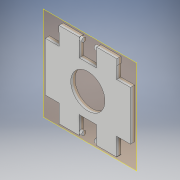
# Autodesk Inventor part: 20_Cube_Insert_focusing_holder_v3
Saved by Autodesk Inventor 2019 (Build 230136000, 136)
## iProperties
Created: 2021-04-22
Part Number: 20_Cube_Insert_focusing_holder_v3
Material: Generic
Document SubType Name: Modeling
Designer: UC2
Density: 1 g/cm^3
Appearance: Default
Author: UC2
Autodesk Inventor part; units mm, degrees
ref_plane "YZ Plane" through (0, 0, 0) normal (1, 0, 0) x (0, 1, 0)
ref_plane "XZ Plane" through (0, 0, 0) normal (0, 1, 0) x (-1, 0, 0)
ref_plane "XY Plane" through (0, 0, 0) normal (0, 0, 1) x (1, 0, 0)
sketch "Skizze1" plane through (0, 0, 0) normal (0, 0, 1) x (1, 0, 0)
  line L0 (0, -42.3366) -> (0, 42.3366) construction
  line L1 (-38.4382, 0) -> (56.3005, 0) construction
  line L2 (0, 0) -> (30.2404, 30.2404) construction
  line L3 (0, 0) -> (42.7664, 0) construction
  line L4 (0, 24.9041) -> (16.9, 24.9041)
  line L5 (16.9, 24.9041) -> (16.9, 21.2841)
  line L6 (16.9, 21.2841) -> (19.092, 19.092)
  line L7 (24.9041, 0) -> (24.9041, 16.9)
  line L8 (24.9041, 16.9) -> (21.2841, 16.9)
  line L9 (21.2841, 16.9) -> (19.092, 19.092)
  line L10 (0, 24.9041) -> (-16.9, 24.9041)
  line L11 (-16.9, 24.9041) -> (-16.9, 21.2841)
  line L12 (-16.9, 21.2841) -> (-19.092, 19.092)
  line L13 (-24.9041, 0) -> (-24.9041, 16.9)
  line L14 (-24.9041, 16.9) -> (-21.2841, 16.9)
  line L15 (-21.2841, 16.9) -> (-19.092, 19.092)
  line L16 (0, 0) -> (30.2404, -30.2404) construction
  line L17 (0, -24.9041) -> (16.9, -24.9041)
  line L18 (16.9, -24.9041) -> (16.9, -21.2841)
  line L19 (16.9, -21.2841) -> (19.092, -19.092)
  line L20 (24.9041, 0) -> (24.9041, -16.9)
  line L21 (24.9041, -16.9) -> (21.2841, -16.9)
  line L22 (21.2841, -16.9) -> (19.092, -19.092)
  line L23 (0, -24.9041) -> (-16.9, -24.9041)
  line L24 (-16.9, -24.9041) -> (-16.9, -21.2841)
  line L25 (-16.9, -21.2841) -> (-19.092, -19.092)
  line L26 (-24.9041, 0) -> (-24.9041, -16.9)
  line L27 (-24.9041, -16.9) -> (-21.2841, -16.9)
  line L28 (-21.2841, -16.9) -> (-19.092, -19.092)
  circle A0 centre (0, 0) radius 10
  dimension "d0" = 45
  dimension "d1" = 16.9
  dimension "d2" = 3.1
  dimension "d3" = 3.62
  dimension "d4" = 20
  constraints: 54 end point, 21 symmetric about line, 3 point on line, 2 horizontal, 2 perpendicular, 1 centre point, 1 coincident, 1 equal length
  measures "d0" angle of L3 L2
  measures "d1" distance of L4.start L4.end
  measures "d2" distance of L5.end L6.end
  measures "d3" distance of L4.end L5.end
  measures "d4" diameter of A0
extrude "Extrusion1" add sketch "Skizze1" along normal blind 2.5
sketch "Skizze2" plane through (0, 0, 2.5) normal (0, 0, 1) x (1, 0, 0)
  line L0 (17.3243, 16.97) -> (5, 16.97) construction
  line L1 (17.3243, 16.97) -> (17.3243, 14.47) construction
  line L2 (5, 14.47) -> (17.3243, 14.47) construction
  line L3 (5, 16.97) -> (5, 14.47) construction
  line L4 (-5, 16.97) -> (-17.3243, 16.97) construction
  line L5 (-5, 16.97) -> (-5, 14.47) construction
  line L6 (-17.3243, 14.47) -> (-5, 14.47) construction
  line L7 (-17.3243, 16.97) -> (-17.3243, 14.47) construction
  circle A0 centre (0, 0) radius 10 construction
  line L8 (16.9, 24.9041) -> (-16.9, 24.9041) construction
  line L9 (-16.9, 24.9041) -> (-16.9, 21.2841) construction
  line L10 (-16.9, 21.2841) -> (-21.2841, 16.9) construction
  line L11 (-21.2841, 16.9) -> (-24.9041, 16.9) construction
  line L12 (-24.9041, 16.9) -> (-24.9041, -16.9) construction
  line L13 (-24.9041, -16.9) -> (-21.2841, -16.9) construction
  line L14 (-21.2841, -16.9) -> (-16.9, -21.2841) construction
  line L15 (-16.9, -21.2841) -> (-16.9, -24.9041) construction
  line L16 (-16.9, -24.9041) -> (16.9, -24.9041) construction
  line L17 (16.9, -24.9041) -> (16.9, -21.2841) construction
  line L18 (16.9, -21.2841) -> (21.2841, -16.9) construction
  line L19 (21.2841, -16.9) -> (24.9041, -16.9) construction
  line L20 (24.9041, -16.9) -> (24.9041, 16.9) construction
  line L21 (24.9041, 16.9) -> (21.2841, 16.9) construction
  line L22 (21.2841, 16.9) -> (16.9, 21.2841) construction
  line L23 (16.9, 21.2841) -> (16.9, 24.9041) construction
  line L24 (-5, 14.47) -> (5, 14.47) construction
  line L25 (5, 14.47) -> (5, 24.9041) construction
  line L26 (5, 24.9041) -> (-5, 24.9041) construction
  line L27 (-5, 24.9041) -> (-5, 14.47) construction
  line L28 (-16.9, 21.2841) -> (-21.2841, 16.9) construction
  line L29 (-16.9, 21.2841) -> (-24.9041, 21.2841) construction
  line L30 (-24.9041, 21.2841) -> (-24.9041, 14.47) construction
  line L31 (-24.9041, 14.47) -> (-16.9, 14.47) construction
  line L32 (-16.9, 14.47) -> (-16.9, 21.2841) construction
  line L33 (0, -34.8857) -> (0, 34.9857) construction
  line L34 (-24.9041, 16.9) -> (-24.9041, -16.9) construction
  line L35 (17.3243, 16.97) -> (17.3243, 14.47) construction
  line L36 (16.9, 21.2841) -> (21.2841, 16.9) construction
  line L37 (21.2841, 16.9) -> (24.9041, 16.9) construction
  line L38 (16.9, 21.2841) -> (21.2841, 16.9) construction
  line L39 (16.9, 21.2841) -> (24.9041, 21.2841) construction
  line L40 (24.9041, 21.2841) -> (24.9041, 14.47) construction
  line L41 (24.9041, 14.47) -> (16.9, 14.47) construction
  line L42 (16.9, 14.47) -> (16.9, 21.2841) construction
  line L43 (16.8, 14.37) -> (25.0041, 14.37)
  line L44 (25.0041, 14.37) -> (25.0041, 21.3841)
  line L45 (25.0041, 21.3841) -> (16.8, 21.3841)
  line L46 (16.8, 21.3841) -> (16.8, 14.37)
  line L47 (-16.8, 14.37) -> (-25.0041, 14.37)
  line L48 (-25.0041, 14.37) -> (-25.0041, 21.3841)
  line L49 (-25.0041, 21.3841) -> (-16.8, 21.3841)
  line L50 (-16.8, 21.3841) -> (-16.8, 14.37)
  line L51 (16.9, 24.9041) -> (-16.9, 24.9041) construction
  line L52 (-5, 14.47) -> (5, 14.47) construction
  line L53 (5, 14.47) -> (5, 24.9041) construction
  line L54 (5, 24.9041) -> (-5, 24.9041) construction
  line L55 (-5, 24.9041) -> (-5, 14.47) construction
  line L56 (5.1, 25.0041) -> (5.1, 14.37)
  line L57 (5.1, 14.37) -> (-5.1, 14.37)
  line L58 (-5.1, 14.37) -> (-5.1, 25.0041)
  line L59 (-5.1, 25.0041) -> (5.1, 25.0041)
  dimension "d8" = 0.1
  dimension "d9" = 0.1
  dimension "d15" = 10
  dimension "d16" = 0.1
  constraints: 64 end point, 10 parallel, 5 perpendicular, 3 horizontal, 3 point on line, 3 symmetric about line, 2 collinear, 10 other
  measures "d8" distance between parallel lines of L41 L43
  measures "d9" distance between parallel lines of L31 L47
  measures "d15" distance between parallel lines of L55 L53
  measures "d16" distance between parallel lines of L53 L56
extrude "Extrusion2" cut sketch "Skizze2" against normal through all
sketch "Skizze3" plane through (0, 0, 2.5) normal (0, 0, 1) x (1, 0, 0)
  line L0 (16.8, 21.3841) -> (16.9, 21.3841) construction
  line L1 (16.9, 21.3841) -> (16.9, 24.9041) construction
  line L2 (-5.1, 24.9041) -> (-16.9, 24.9041) construction
  line L3 (16.9, 24.9041) -> (5.1, 24.9041) construction
  line L4 (-16.9, 24.9041) -> (-16.9, 21.3841) construction
  line L5 (-16.9, 21.3841) -> (-16.8, 21.3841) construction
  line L6 (-16.8, 21.3841) -> (-16.8, 14.37) construction
  line L7 (-16.8, 14.37) -> (-24.9041, 14.37) construction
  line L8 (-24.9041, 14.37) -> (-24.9041, -16.9) construction
  line L9 (-24.9041, -16.9) -> (-21.2841, -16.9) projected
  line L10 (-21.2841, -16.9) -> (-16.9, -21.2841) projected
  line L11 (-16.9, -21.2841) -> (-16.9, -24.9041) projected
  line L12 (-16.9, -24.9041) -> (16.9, -24.9041) construction
  line L13 (16.9, -24.9041) -> (16.9, -21.2841) projected
  line L14 (16.9, -21.2841) -> (21.2841, -16.9) projected
  line L15 (21.2841, -16.9) -> (24.9041, -16.9) projected
  line L16 (24.9041, -16.9) -> (24.9041, 14.37) construction
  line L17 (24.9041, 14.37) -> (16.8, 14.37) construction
  line L18 (16.8, 14.37) -> (16.8, 21.3841) construction
  circle A0 centre (0, 0) radius 10 construction
  line L19 (24.8041, -16.8) -> (21.2426, -16.8)
  line L20 (21.2426, -16.8) -> (16.8, -21.2426)
  line L21 (16.8, -21.2426) -> (16.8, -24.8041)
  line L22 (16.8, -24.8041) -> (-16.8, -24.8041) construction
  line L23 (-16.8, -24.8041) -> (-16.8, -21.2426)
  line L24 (-16.8, -21.2426) -> (-21.2426, -16.8)
  line L25 (-21.2426, -16.8) -> (-24.8041, -16.8)
  line L26 (-24.8041, -16.8) -> (-24.8041, 14.27) construction
  line L27 (-24.8041, 14.27) -> (-16.7, 14.27) construction
  line L28 (-16.7, 14.27) -> (-16.7, 21.4841) construction
  line L29 (-16.7, 21.4841) -> (-16.8, 21.4841) construction
  line L30 (-16.8, 21.4841) -> (-16.8, 24.8041) construction
  line L31 (-16.8, 24.8041) -> (-2.7, 24.8041) construction
  line L32 (-2.7, 24.8041) -> (-2.7, 14.27) construction
  line L33 (-2.7, 14.27) -> (2.7, 14.27) construction
  line L34 (2.7, 14.27) -> (2.7, 24.8041) construction
  line L35 (2.7, 24.8041) -> (16.8, 24.8041) construction
  line L36 (16.8, 24.8041) -> (16.8, 21.4841) construction
  line L37 (16.8, 21.4841) -> (16.7, 21.4841) construction
  line L38 (16.7, 21.4841) -> (16.7, 14.27) construction
  line L39 (16.7, 14.27) -> (24.8041, 14.27) construction
  line L40 (24.8041, 14.27) -> (24.8041, -16.8) construction
  line L41 (-24.8041, -16.8) -> (-24.8041, -16.9)
  line L42 (-16.8, -24.8041) -> (-16.9, -24.8041)
  line L43 (16.8, -24.8041) -> (16.9, -24.8041)
  line L44 (24.8041, -16.8) -> (24.8041, -16.9)
  line L45 (5.1, 24.9041) -> (5.1, 14.37) projected
  line L46 (5.1, 14.37) -> (-5.1, 14.37) projected
  line L47 (-5.1, 14.37) -> (-5.1, 24.9041) projected
  dimension "d12" = 0.1
  constraints: 52 end point, 5 point on line, 2 perpendicular, 1 parallel, 17 other
  measures "d12" distance between parallel lines of L15 L19
extrude "Extrusion3" cut sketch "Skizze3" against normal up to surface (2.5 mm away)
mirror "Spiegeln1" about plane through (0, 0, 0) normal (0, 1, 0) of "Extrusion2"
ref_plane "Arbeitsebene1" through (0, 0, 1.25) normal (0, 0, 1) x (1, 0, 0)
sketch "Skizze4" plane through (0, 0, 2.5) normal (0, 0, 1) x (1, 0, 0)
  circle A0 centre (0, 0) radius 10 construction
  line L0 (-24.9041, -14.37) -> (-16.8, -14.37) construction
  line L1 (-16.8, -14.37) -> (-16.8, -24.8041) construction
  line L2 (-16.8, -24.8041) -> (-16.9, -24.8041) construction
  line L3 (-16.9, -24.8041) -> (-16.9, -24.9041) construction
  line L4 (-16.9, -24.9041) -> (-5.1, -24.9041) construction
  line L5 (-5.1, -24.9041) -> (-5.1, -14.37) construction
  line L6 (-5.1, -14.37) -> (5.1, -14.37) construction
  line L7 (5.1, -14.37) -> (5.1, -24.9041) construction
  line L8 (5.1, -24.9041) -> (16.9, -24.9041) construction
  line L9 (16.9, -24.9041) -> (16.9, -24.8041) construction
  line L10 (16.9, -24.8041) -> (16.8, -24.8041) construction
  line L11 (16.8, -24.8041) -> (16.8, -14.37) construction
  line L12 (16.8, -14.37) -> (24.9041, -14.37) construction
  line L13 (24.9041, -14.37) -> (24.9041, 14.37) construction
  line L14 (24.9041, 14.37) -> (16.8, 14.37) construction
  line L15 (16.8, 14.37) -> (16.8, 21.3841) construction
  line L16 (16.8, 21.3841) -> (16.9, 21.3841) construction
  line L17 (16.9, 21.3841) -> (16.9, 24.9041) construction
  line L18 (16.9, 24.9041) -> (5.1, 24.9041) construction
  line L19 (5.1, 24.9041) -> (5.1, 14.37) construction
  line L20 (5.1, 14.37) -> (-5.1, 14.37) construction
  line L21 (-5.1, 14.37) -> (-5.1, 24.9041) construction
  line L22 (-5.1, 24.9041) -> (-16.9, 24.9041) construction
  line L23 (-16.9, 24.9041) -> (-16.9, 21.3841) construction
  line L24 (-16.9, 21.3841) -> (-16.8, 21.3841) construction
  line L25 (-16.8, 21.3841) -> (-16.8, 14.37) construction
  line L26 (-16.8, 14.37) -> (-24.9041, 14.37) construction
  line L27 (-24.9041, 14.37) -> (-24.9041, -14.37) construction
  line L28 (5.1, 24.9041) -> (3.6, 24.9041)
  line L29 (3.6, 24.9041) -> (3.6, 22.4041)
  line L30 (3.6, 22.4041) -> (5.1, 22.4041)
  line L31 (5.1, 22.4041) -> (5.1, 24.9041)
  line L32 (-34.8657, 0) -> (34.8657, 0) construction
  line L33 (0, 34.8657) -> (0, -34.8657) construction
  line L34 (5.1, -24.9041) -> (3.6, -24.9041)
  line L35 (3.6, -24.9041) -> (3.6, -22.4041)
  line L36 (3.6, -22.4041) -> (5.1, -22.4041)
  line L37 (5.1, -22.4041) -> (5.1, -24.9041)
  line L38 (-5.1, 24.9041) -> (-3.6, 24.9041)
  line L39 (-3.6, 24.9041) -> (-3.6, 22.4041)
  line L40 (-3.6, 22.4041) -> (-5.1, 22.4041)
  line L41 (-5.1, 22.4041) -> (-5.1, 24.9041)
  line L42 (-3.6, -22.4041) -> (-5.1, -22.4041)
  line L43 (-3.6, -24.9041) -> (-3.6, -22.4041)
  line L44 (-5.1, -24.9041) -> (-3.6, -24.9041)
  line L45 (-5.1, -22.4041) -> (-5.1, -24.9041)
  dimension "d18" = 2.5
  dimension "d19" = 1.5
  constraints: 32 end point, 9 symmetric about line, 2 parallel, 1 horizontal, 1 perpendicular
  measures "d18" distance of L28.end L29.end
  measures "d19" distance of L18.end L28.end
extrude "Extrusion4" add sketch "Skizze4" against normal up to surface (2.5 mm away)
sketch "Skizze5" plane through (3.6, 22.4041, 2.5) normal (-1, 0, 0) x (0, 0, 1)
  line L0 (-2.5, 0) -> (-2.5, 2.5) construction
  line L1 (0, 0) -> (-2.5, 0) construction
  line L2 (0, 2.5) -> (0, 0) construction
  line L3 (0, 2.5) -> (-2.5, 2.5) construction
  circle A0 centre (-1.25, 1.25) radius 1.25
  line L4 (-1.25, 12.4616) -> (-1.25, -57.2697) projected
  line L5 (0, 2.5) -> (-2.5, 2.5)
  line L6 (-2.5, 2.5) -> (-2.5, 0)
  line L7 (-2.5, 0) -> (0, 0)
  line L8 (0, 0) -> (0, 2.5)
  point P0 (-2.5, -22.4041)
  constraints: 8 end point, 2 parallel, 2 tangent, 1 centre point, 1 horizontal, 1 perpendicular, 1 point on line
extrude "Extrusion5" cut sketch "Skizze5" against normal up to surface (1.5 mm away) contours L8 L7 A0 | A0 L5 L8 | A0 L6 L5 | L7 L6 A0
mirror "Spiegeln2" about plane through (0, 0, 0) normal (0, 1, 0) of "Extrusion5"
mirror "Spiegeln3" about plane through (0, 0, 0) normal (1, 0, 0) of "Extrusion5", "Spiegeln2"
